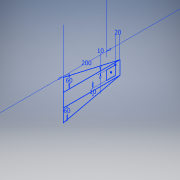
# Autodesk Inventor part: Motor Mount_2
Saved by Autodesk Inventor 2018 (Build 220112000, 112)
## iProperties
Created: 2018-11-09
Part Number: Motor Mount_2
Material: Generic
Document SubType Name: Modeling
Designer: Cameron
Density: 1 g/cm^3
Appearance: Default
Author: Cameron
Autodesk Inventor part; units mm, degrees
ref_plane "YZ Plane" through (0, 0, 0) normal (1, 0, 0) x (0, 1, 0)
ref_plane "XZ Plane" through (0, 0, 0) normal (0, 1, 0) x (-1, 0, 0)
ref_plane "XY Plane" through (0, 0, 0) normal (0, 0, 1) x (1, 0, 0)
ref_plane "Work Plane1" through (0, 0, 0) normal (0, 0, 1) x (1, 0, 0)
sketch "Sketch1" plane through (0, 0, 0) normal (0, 0, 1) x (1, 0, 0)
  line L0 (2, -42.3) -> (0, -40.3) projected
  line L1 (2, -42.3) -> (40.3, -42.3) projected
  line L2 (42.3, -40.3) -> (40.3, -42.3) projected
  line L3 (42.3, -2) -> (42.3, -40.3) projected
  line L4 (40.3, 0) -> (42.3, -2) projected
  line L5 (2, 0) -> (40.3, 0) projected
  line L6 (0, -2) -> (2, 0) projected
  line L7 (0, -2) -> (0, -40.3) projected
  circle A0 centre (21.15, -21.15) radius 1.95 projected
  line L8 (-10, 20) -> (52.3, 20)
  line L9 (52.3, 20) -> (52.3, -240)
  line L10 (52.3, -240) -> (-10, -240)
  line L11 (-10, -240) -> (-10, 20)
  line L12 (52.3, 20) -> (92.3, -240)
  line L13 (92.3, -240) -> (52.3, -240)
  line L14 (-10, -240) -> (-50, -240)
  line L15 (-50, -240) -> (-10, 20)
  point P0 (0, 0)
  dimension "d0" = 20
  dimension "d1" = 260
  dimension "d2" = 10
  dimension "d3" = 10
  dimension "d4" = 40
  dimension "d5" = 40
  constraints: 16 end point, 2 horizontal, 2 parallel, 1 perpendicular, 1 point on line
  measures "d0" distance between parallel lines of L8 L5
  measures "d1" distance between parallel lines of L8 L10
  measures "d2" distance between parallel lines of L11 L7
  measures "d3" distance between parallel lines of L9 L3
  measures "d4" distance of L12.end L9.end
  measures "d5" distance of L10.end L14.end
extrude "Extrusion1" add sketch "Sketch1" against normal blind 10 contours L8 L9 L10 L11 | L11 L14 L15 | L12 L13 L9
fillet "Fillet1" radius 2 5 edges at (-30, -110, 0) (21.15, 20, 0) (72.3, -110, 0) (52.3, 20, -5) (-10, 20, -5)
ref_plane "Work Plane2" through (0, 0, -45) normal (0, 0, -1) x (-1, 0, 0)
sketch "Sketch4" plane through (0, 0, -45) normal (0, 0, -1) x (-1, 0, 0)
  arc A0 (-50.5842, 20) -> (-52.5609, 18.3041) centre (-50.5842, 18) ccw projected
  line L0 (-52.5609, 18.3041) -> (-92.3, -240) projected
  line L1 (-92.3, -240) -> (50, -240) projected
  line L2 (50, -240) -> (10.2609, 18.3041) projected
  arc A1 (10.2609, 18.3041) -> (8.2842, 20) centre (8.2842, 18) ccw projected
  line L3 (8.2842, 20) -> (-50.5842, 20) projected
  line L4 (-2, -42.3) -> (-40.3, -42.3) projected
  line L5 (-40.3, -42.3) -> (-42.3, -40.3) projected
  line L6 (-42.3, -40.3) -> (-42.3, -2) projected
  line L7 (-42.3, -2) -> (-40.3, 0) projected
  line L8 (-40.3, 0) -> (-2, 0) projected
  line L9 (-2, 0) -> (0, -2) projected
  line L10 (0, -2) -> (0, -40.3) projected
  line L11 (0, -40.3) -> (-2, -42.3) projected
  circle A2 centre (-21.15, -21.15) radius 18 projected
  point P0 (0, 0)
extrude "Extrusion3" add sketch "Sketch4" along normal blind 10 contours L3 A1 L2 L1 L0 A0 | L4 L5 L6 L7 L8 L9 L10 L11
body "Solid1"
